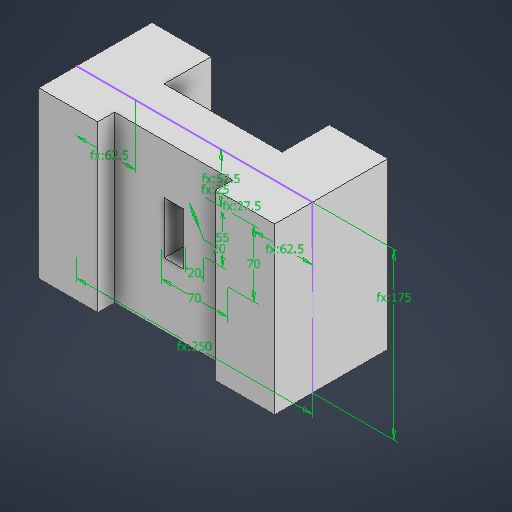
# Autodesk Inventor part: Part3
Saved by Autodesk Inventor 2027.1 (Build 311270010, 270A)
## iProperties
Created: 2026-09-28
Part Number: Part3
Material: Generic
Document SubType Name: Modeling
Designer: daniel
Density: 1 g/cm^3
Appearance: Default
Author: daniel
Autodesk Inventor part; units mm, degrees
ref_plane "YZ Plane" through (0, 0, 0) normal (1, 0, 0) x (0, 1, 0)
ref_plane "XZ Plane" through (0, 0, 0) normal (0, 1, 0) x (-1, 0, 0)
ref_plane "XY Plane" through (0, 0, 0) normal (0, 0, 1) x (1, 0, 0)
sketch "Sketch1" plane through (0, 0, 0) normal (0, 0, 1) x (1, 0, 0)
  line L0 (-117.1316, 93.6595) -> (132.8684, 93.6595)
  line L1 (132.8684, 93.6595) -> (132.8684, -81.3405)
  line L2 (132.8684, -81.3405) -> (-117.1316, -81.3405)
  line L3 (-117.1316, -81.3405) -> (-117.1316, 93.6595)
  line L4 (-54.6316, 93.6595) -> (-54.6316, -81.3405)
  line L5 (70.3684, 93.6595) -> (70.3684, -81.3405)
  line L6 (-27.1316, 41.1595) -> (42.8684, 41.1595)
  line L7 (42.8684, 41.1595) -> (42.8684, -28.8405)
  line L8 (42.8684, -28.8405) -> (-27.1316, -28.8405)
  line L9 (-27.1316, -28.8405) -> (-27.1316, 41.1595)
  circle A0 centre (7.8684, 18.6595) radius 10
  line L10 (-2.1316, 41.1595) -> (17.8684, 41.1595)
  line L11 (17.8684, 41.1595) -> (17.8684, -13.8405)
  line L12 (17.8684, -13.8405) -> (-2.1316, -13.8405)
  line L13 (-2.1316, -13.8405) -> (-2.1316, 41.1595)
  point P0 (17.8684, 41.1595)
  point P1 (17.8684, 18.6595)
  point P2 (-2.1316, 18.6595)
  dimension "d0" = 250
  dimension "d1" = 175
  dimension "d2" = 62.5
  dimension "d3" = 62.5
  dimension "d8" = 70
  dimension "d9" = 70
  dimension "d10" = 52.5
  dimension "d11" = 27.5
  dimension "d12" = 20
  dimension "d19" = 20
  dimension "d20" = 55
  dimension "d21" = 25
  constraints: 28 end point, 6 parallel, 5 perpendicular, 5 point on line, 3 horizontal, 1 centre point
  measures "d0" distance of L1.end L2.end
  measures "d1" distance of L0.end L1.end
  measures "d2" distance between parallel lines of L1 L5
  measures "d3" distance between parallel lines of L3 L4
  measures "d8" distance of L7.end L8.end
  measures "d9" distance of L6.end L7.end
  measures "d10" distance between parallel lines of L0 L6
  measures "d11" distance between parallel lines of L5 L7
  measures "d12" diameter of A0
  measures "d19" distance of L11.end L12.end
  measures "d20" distance of L10.end L11.end
  measures "d21" distance between parallel lines of L7 L11
extrude "Extrusion1" add sketch "Sketch1" along normal blind 40 and the other way blind 80 contours L0 L4 L2 L3 | L0 L1 L2 L5
extrude "Extrusion2" add sketch "Sketch1" along normal blind 22 and the other way blind 80 contours L0 L5 L2 L4 | L6 L13 L12 L11 L7 L8 L9 | L6 L11 A0 L13 | A0 | A0 L11 L12 L13
extrude "Extrusion3" cut sketch "Sketch1" along normal blind 22 and the other way blind 3 contours L6 L11 A0 L13 | A0 | A0 L11 L12 L13
extrude "Extrusion4" cut sketch "Sketch1" against normal blind 25 contours A0
sketch "Sketch3" plane through (-117.1316, -81.3405, -80) normal (0, -1, 0) x (1, 0, 0)
  line L0 (0, 0) -> (250, 0) projected
  line L1 (62.8423, 0) -> (187.8423, 0)
  line L2 (187.8423, 0) -> (187.8423, 50)
  line L3 (187.8423, 50) -> (62.8423, 50)
  line L4 (62.8423, 50) -> (62.8423, 0)
  point P0 (117.1316, 80)
  dimension "d22" = 125
  dimension "d23" = 50
  constraints: 8 end point, 2 parallel, 1 horizontal, 1 perpendicular, 1 point on line
  measures "d22" distance of L3.end L2.end
  measures "d23" distance of L2.end L1.end
extrude "Extrusion5" cut sketch "Sketch3" against normal through all
equation "\"d0\" = 5 * Product_dia"
equation "\"d1\" = 3.5 * Product_dia"
equation "\"d2\" = 0.25 * d0"
equation "\"d3\" = d2"
equation "\"d10\" = -0.5 * d9 + 0.5 * d1"
equation "\"d11\" = -0.5 * d8 + 0.5 * d0 - d2"
equation "\"d21\" = -0.5 * d19 + 0.5 * d8"
equation "\"ProductBaseHeight\" = 35"
equation "\"GridClearance\" = 3"
equation "\"GridBorderThickness\" = 5"
equation "\"GridTotalSize\" = 63"
equation "\"GridBorderFillets\" = 7"
equation "\"BaseTotalWidth\" = 352"
equation "\"GridProcutClearance\" = 3"
equation "\"Product_dia\" = 50"
body "Solid1"
